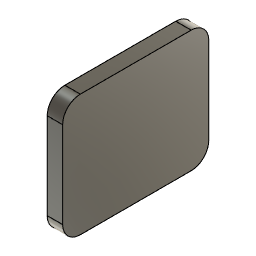
7.1 boundry fill (Autodesk Fusion 360 design; units mm, degrees)
Autodesk Fusion 360 part; units mm, degrees
sketch "Sketch1" plane through (0, 0, 0) normal (1, 0, 0) x (0, 1, 0)
  circle A0 centre (0, 0) radius 45
  line L0 (-1.7761, 24.4773) -> (-1.7761, 15.686)
  line L1 (0.9712, 24.4773) -> (0.9712, 15.686)
  line L2 (-4.7479, 40.7242) -> (-4.7479, 37.8324)
  line L3 (-4.7479, 37.8324) -> (-1.6597, 37.8324)
  line L4 (-1.6597, 37.8324) -> (-1.6597, 34.0517)
  line L5 (-1.6597, 34.0517) -> (1.3885, 34.0517)
  line L6 (1.3885, 34.0517) -> (1.3885, 37.8324)
  line L7 (1.3885, 37.8324) -> (4.7125, 37.8324)
  line L8 (4.7125, 37.8324) -> (4.7125, 40.7283)
  line L9 (-6.6829, 7.2287) -> (-3.6696, 6.0858)
  line L10 (-3.6696, 6.0858) -> (-17.3847, -37.1318)
  line L11 (-17.7596, -36.954) -> (-16.1385, -25.606)
  line L12 (-16.1385, -25.606) -> (-6.6829, 7.2287)
  line L13 (0, 0) -> (0, -12.4098) construction
  line L14 (16.1385, -25.606) -> (6.6829, 7.2287)
  line L15 (3.6696, 6.0858) -> (17.3847, -37.1318)
  line L16 (6.6829, 7.2287) -> (3.6696, 6.0858)
  line L17 (17.7596, -36.954) -> (16.1385, -25.606)
  line L18 (15.1489, -14.4423) -> (17.5326, -21.9534)
  line L19 (19.4017, -21.3603) -> (16.9104, -13.7134)
  arc A1 (16.9561, -13.8536) -> (15.1489, -14.4423) centre (16.0297, -14.0779) ccw
  arc A2 (17.5326, -21.9534) -> (19.397, -21.346) centre (18.4671, -21.6568) ccw
  arc A3 (-9.6373, 17.866) -> (8.8324, 17.866) centre (-0.4024, 20.0816) ccw
  arc A4 (8.9914, 21.4775) -> (-9.7962, 21.4775) centre (-0.4024, 20.0816) ccw
  arc A5 (-12.0223, 17.866) -> (11.2175, 17.866) centre (-0.4024, 20.0816) ccw
  arc A6 (11.3442, 21.4775) -> (-12.149, 21.4775) centre (-0.4024, 20.0816) ccw
  line L20 (-12.149, 21.4775) -> (-9.7962, 21.4775)
  line L21 (-9.6373, 17.866) -> (-12.0223, 17.866)
  line L22 (11.2175, 17.866) -> (8.8324, 17.866)
  line L23 (8.9914, 21.4775) -> (11.3442, 21.4775)
  arc A7 (-1.7761, 24.4773) -> (-1.7761, 15.686) centre (-0.4024, 20.0816) ccw
  arc A8 (0.9712, 15.686) -> (0.9712, 24.4773) centre (-0.4024, 20.0816) ccw
  circle A9 centre (0, 0) radius 41
  dimension "d1" = 90
  dimension "d2" = 82
  constraint coincident A0.centre L13.start
  constraint concentric A0 A9
  constraint concentric A3 A5
  constraint concentric A5 A7
  constraint vertical L0
  constraint coincident L1.end A7
  constraint parallel L0 L1
  constraint parallel L1 L2
  constraint perpendicular L2 L3
  constraint perpendicular L3 L4
  constraint perpendicular L4 L5
  constraint perpendicular L5 L6
  constraint perpendicular L6 L7
  constraint perpendicular L5 L8
  constraint vertical L13
  constraint symmetric L9.start L13 L14.end
  constraint symmetric L9.end L13 L15.start
  constraint symmetric L11.end L13 L14.start
  constraint parallel L15 L18
  constraint coincident L19.end A1
  constraint coincident L19.start A2
  constraint coincident L19 A1.start
  constraint coincident L19 A2.end
  constraint coincident L10.end A9
  constraint horizontal L20
  constraint coincident A6.start A5
  constraint coincident A3.start L22
  constraint coincident A4.start L20
  constraint concentric A3 A4
  constraint concentric A5 A6
  constraint collinear L21 L22
  constraint concentric A7 A8
  constraint coincident L2.start A9
  constraint coincident L8.end A9
  constraint coincident L17.start A9
  constraint coincident L15.end A9
  constraint horizontal L23
  constraint horizontal L22
  measures "d1" diameter of A0
  measures "d2" diameter of A9
extrude "Extrude1" add sketch "Sketch1" along normal blind 10 contours A0 makes body 1
extrude "Extrude2" add sketch "Sketch1" along normal blind 6 contours L2 L3 L4 L5 L6 L7 L8 L9 L10 L11 L12 L14 L15 L16 L17 A9 bodies 1
fillet "Fillet1" radius 1.6 2 edges at (10, -38.2254, 14.8262) (10, -41.9547, -16.2727) on bodies 1
sketch "Sketch2" plane through (0, 0, 0) normal (1, 0, 0) x (0, 1, 0)
  line L0 (-68.9346, 55.3313) -> (70.9942, 55.3313)
  line L1 (70.9942, 55.3313) -> (70.9942, -61.2761)
  line L2 (70.9942, -61.2761) -> (-68.9346, -61.2761)
  line L3 (-68.9346, -61.2761) -> (-68.9346, 55.3313)
  constraint horizontal L0
  constraint vertical L1
  constraint horizontal L2
  constraint vertical L3
extrude "Extrude3" add sketch "Sketch2" along normal blind 14.803 separate body makes body 2
combine "Combine1" operation cut target body 2 tool bodies 1
fillet "Fillet2" radius 16.884 4 edges at (7.4015, 70.9942, -61.2761) (7.4015, 70.9942, 55.3313) (7.4015, -68.9346, -61.2761) (7.4015, -68.9346, 55.3313) on bodies 2
